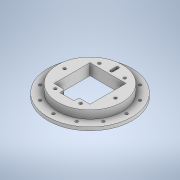
# Autodesk Inventor part: Chasis
Saved by Autodesk Inventor 2022 (Build 260153000, 153)
## iProperties
Created: 2022-02-26
Part Number: Chasis
Material: Genérico
Document SubType Name: Modeling
Designer: JK
Density: 1 g/cm^3
Appearance: Valor por defecto
Author: JK
Autodesk Inventor part; units mm, degrees
ref_plane "YZ Plane" through (0, 0, 0) normal (1, 0, 0) x (0, 1, 0)
ref_plane "XZ Plane" through (0, 0, 0) normal (0, 1, 0) x (-1, 0, 0)
ref_plane "XY Plane" through (0, 0, 0) normal (0, 0, 1) x (1, 0, 0)
sketch "Boceto1" plane through (0, 0, 0) normal (0, 1, 0) x (-1, 0, 0)
  line L0 (-21.7, 21.7) -> (21.7, 21.7)
  line L1 (21.7, 21.7) -> (21.7, -21.7)
  line L2 (21.7, -21.7) -> (-21.7, -21.7)
  line L3 (-21.7, -21.7) -> (-21.7, 21.7)
  line L4 (-21.7, 21.7) -> (21.7, -21.7) construction
  line L5 (21.7, 21.7) -> (-21.7, -21.7) construction
  circle A0 centre (0, 0) radius 39
  dimension "d0" = 43.4
  dimension "d1" = 43.4
  dimension "d2" = 78
  constraints: 12 end point, 2 midpoint, 2 parallel, 1 centre point, 1 coincident, 1 horizontal, 1 perpendicular
  measures "d0" distance of L0.end L1.end
  measures "d1" distance of L1.end L2.end
  measures "d2" diameter of A0
extrude "Extrusión1" add sketch "Boceto1" along normal blind 5.63
sketch "Boceto2" plane through (0, 5.63, 0) normal (0, 1, 0) x (1, 0, 0)
  circle A0 centre (-26, -15.0111) radius 2.15
  line L0 (0, 0) -> (-31.4817, 0)
  line L1 (0, 0) -> (-26, -15.0111)
  circle A1 centre (-26, 15.011) radius 2.15
  circle A2 centre (26, -15.0112) radius 2.15
  circle A3 centre (26, 15.0111) radius 2.15
  line L2 (26, 15.0111) -> (-26, -15.0111)
  line L3 (26, -15.0112) -> (-26, 15.011)
  circle A4 centre (0, 0) radius 39 projected
  line L4 (21.7, -21.7) -> (-21.7, -21.7) projected
  line L5 (-21.7, -21.7) -> (-21.7, 21.7) projected
  line L6 (-21.7, 21.7) -> (21.7, 21.7) projected
  line L7 (21.7, 21.7) -> (21.7, -21.7) projected
  dimension "d5" = 4.3
  dimension "d6" = 30
  dimension "d7" = 26
  dimension "d10" = 26
  dimension "d11" = 30
  dimension "d12" = 26
  dimension "d13" = 26
  dimension "d14" = 15.011
  constraints: 8 end point, 4 centre point, 3 equal radius, 1 collinear, 1 horizontal
  measures "d5" diameter of A0
  measures "d6" angle of L0 L1
  measures "d7" horizontal distance of L0.start L1.end
  measures "d10" horizontal distance of L3.end L0.start
  measures "d11" angle of L0 L3
  measures "d12" horizontal distance of L2.start L0.start
  measures "d13" horizontal distance of L0.start L3.start
  measures "d14" vertical distance of L0.start L3.end
extrude "Extrusión2" cut sketch "Boceto2" against normal through all contours A0 | A1 | A2 | A3
sketch "Boceto3" plane through (0, 5.63, 0) normal (0, 1, 0) x (1, 0, 0)
  circle A0 centre (-26, 15.011) radius 2.15 projected
  circle A1 centre (-26, 15.011) radius 4.3
  line L0 (-21.7, -21.7) -> (-21.7, 21.7) projected
  circle A2 centre (26, 15.0111) radius 2.15 projected
  circle A3 centre (26, 15.0111) radius 4.3
  line L1 (21.7, 21.7) -> (21.7, -21.7) projected
  circle A4 centre (26, -15.0112) radius 2.15 projected
  circle A5 centre (26, -15.0112) radius 4.3
  circle A6 centre (-26, -15.0111) radius 2.15 projected
  circle A7 centre (-26, -15.0111) radius 4.3
  circle A8 centre (26, -15.0112) radius 2.15 projected
  circle A9 centre (26, 15.0111) radius 2.15 projected
  circle A10 centre (-26, -15.0111) radius 2.15 projected
  circle A11 centre (-26, 15.011) radius 2.15 projected
  circle A12 centre (0, 0) radius 39 projected
  line L2 (21.7, -21.7) -> (-21.7, -21.7) projected
  line L3 (-21.7, -21.7) -> (-21.7, 21.7) projected
  line L4 (-21.7, 21.7) -> (21.7, 21.7) projected
  line L5 (21.7, 21.7) -> (21.7, -21.7) projected
  point P0 (-21.7, -15.0111)
  point P1 (-21.7, 15.011)
  point P2 (21.7, 15.0111)
  point P3 (21.7, -15.0112)
  constraints: 4 centre point, 4 coincident, 4 tangent
extrude "Extrusión3" add sketch "Boceto3" along normal blind 4 contours A1 | A3 | A5 | A7 | A12
sketch "Boceto5" plane through (0, 9.63, 0) normal (0, 1, 0) x (1, 0, 0)
  circle A0 centre (-30.6, 0) radius 1.65
  point P0 (0, 0)
  dimension "d24" = 3.3
  dimension "d30" = 30.6
  constraints: 1 centre point
  measures "d24" diameter of A0
  measures "d30" distance of point (0, 0) A0.centre
extrude "Extrusión5" cut sketch "Boceto5" against normal through all
pattern_circular "Patrón circular1" count 6 over 360 about axis through (0, 0, 0) along (0, 1, 0) of "Extrusión5"
sketch "Boceto6" plane through (0, 9.63, 0) normal (0, 1, 0) x (1, 0, 0)
  circle A0 centre (0, 33) radius 1.65
  circle A1 centre (0, 26) radius 1.65
  line L0 (-1.65, 33) -> (1.65, 33)
  line L1 (1.65, 33) -> (1.65, 26)
  line L2 (1.65, 26) -> (-1.65, 26)
  line L3 (-1.65, 26) -> (-1.65, 33)
  point P0 (0, 0)
  point P1 (-1.65, 26)
  dimension "d31" = 3.3
  dimension "d32" = 26
  dimension "d33" = 7
  constraints: 8 end point, 3 vertical, 2 parallel, 1 horizontal, 1 perpendicular, 6 other
  measures "d32" distance of point (0, 0) point (0, 26)
  measures "d33" distance of L0.end L1.end
extrude "Extrusión6" cut sketch "Boceto6" against normal blind 10
sketch "Boceto7" plane through (0, 0, 0) normal (0, -1, 0) x (1, 0, 0)
  line L0 (21.7, 21.7) -> (-21.7, 21.7) projected
  line L1 (8.5, 27.7) -> (-8.5, 27.7)
  line L2 (-8.5, 27.7) -> (-8.5, 21.7)
  line L3 (-8.5, 21.7) -> (8.5, 21.7)
  line L4 (8.5, 21.7) -> (8.5, 27.7)
  point P0 (0, 0)
  dimension "d36" = 8.5
  dimension "d37" = 6
  dimension "d38" = 17
  constraints: 8 end point, 2 parallel, 1 horizontal, 1 perpendicular, 1 point on line
  measures "d36" distance from line of point (0, 0) L4
  measures "d37" distance between parallel lines of L0 L1
  measures "d38" distance between parallel lines of L4 L2
extrude "Extrusión7" cut sketch "Boceto7" against normal through all
fillet "Empalme2" radius 2 4 edges at (8.5, 7.63, 21.7) (8.5, 2.815, 21.7) (-8.5, 2.815, 21.7) (-8.5, 7.63, 21.7)
sketch "Boceto8" plane through (0, 0, 0) normal (0, -1, 0) x (1, 0, 0)
  arc A0 (-10.5, 21.7) -> (-8.5, 23.7) centre (-10.5, 23.7) ccw projected
  line L0 (-8.5, 23.7) -> (-8.5, 27.7) projected
  line L1 (-8.5, 27.7) -> (8.5, 27.7) projected
  line L2 (8.5, 27.7) -> (8.5, 23.7) projected
  arc A1 (8.5, 23.7) -> (10.5, 21.7) centre (10.5, 23.7) ccw projected
  line L3 (21.7, 21.7) -> (10.5, 21.7) projected
  line L4 (21.7, -21.7) -> (21.7, 21.7) projected
  line L5 (-21.7, -21.7) -> (21.7, -21.7) projected
  line L6 (-21.7, 21.7) -> (-21.7, -21.7) projected
  line L7 (-10.5, 21.7) -> (-21.7, 21.7) projected
  circle A2 centre (0, 0) radius 39 projected
  circle A3 centre (-26, -15.011) radius 2.15 projected
  circle A4 centre (-26, 15.0111) radius 2.15 projected
  circle A5 centre (26, -15.0111) radius 2.15 projected
  circle A6 centre (26, 15.0112) radius 2.15 projected
  circle A7 centre (-30.6, 0) radius 1.65 projected
  circle A8 centre (-15.3, 26.5004) radius 1.65 projected
  circle A9 centre (15.3, 26.5004) radius 1.65 projected
  circle A10 centre (30.6, 0) radius 1.65 projected
  circle A11 centre (15.3, -26.5004) radius 1.65 projected
  circle A12 centre (-15.3, -26.5004) radius 1.65 projected
  line L8 (-1.65, -33) -> (-1.65, -26) projected
  arc A13 (1.65, -26) -> (-1.65, -26) centre (0, -26) ccw projected
  line L9 (1.65, -26) -> (1.65, -33) projected
  arc A14 (-1.65, -33) -> (1.65, -33) centre (0, -33) ccw projected
  circle A15 centre (0, 0) radius 50.578
  dimension "d42" = 101.156
  constraints: 1 centre point, 1 coincident
  measures "d42" diameter of A15
extrude "Extrusión8" add sketch "Boceto8" along normal blind 4 contours A2 | A15
sketch "Boceto9" plane through (0, 0, 0) normal (0, 1, 0) x (1, 0, 0)
  circle A0 centre (0, -43.944) radius 1.65
  point P0 (0, 0)
  dimension "d45" = 3.3
  dimension "d46" = 43.944
  constraints: 1 centre point
  measures "d45" diameter of A0
  measures "d46" distance of A0.centre point (0, 0)
extrude "Extrusión9" cut sketch "Boceto9" against normal through all
pattern_circular "Patrón circular2" count 12 over 360 about axis through (0, 0, 0) along (0, -1, 0) of "Extrusión9"
sketch "Boceto10" plane through (0, 9.63, 0) normal (0, 1, 0) x (1, 0, 0)
  circle A0 centre (-26, -15.0111) radius 2.15 projected
  circle A1 centre (-26, 15.011) radius 2.15 projected
  circle A2 centre (26, 15.0111) radius 2.15 projected
  circle A3 centre (26, -15.0112) radius 2.15 projected
  point P0 (0, 0)
extrude "Extrusión10" add sketch "Boceto10" against normal up to surface (13.63 mm away)
sketch "Boceto11" plane through (0, -4, 0) normal (0, -1, 0) x (1, 0, 0)
  circle A0 centre (43.944, 0) radius 1.65 projected
  line L0 (46.794, -1.6454) -> (43.944, -3.2909)
  line L1 (43.944, -3.2909) -> (41.094, -1.6454)
  line L2 (41.094, -1.6454) -> (41.094, 1.6454)
  line L3 (41.094, 1.6454) -> (43.944, 3.2909)
  line L4 (43.944, 3.2909) -> (46.794, 1.6454)
  line L5 (46.794, 1.6454) -> (46.794, -1.6454)
  circle A1 centre (43.944, 0) radius 2.85
  point P0 (0, 0)
  dimension "d54" = 5.7
  constraints: 12 end point, 2 coincident, 1 centre point, 1 tangent, 1 vertical alignment, 13 other
  measures "d54" diameter of A1
extrude "Extrusión11" [suppressed]
pattern_circular "Patrón circular3" [suppressed]
sketch "Boceto12" plane through (0, -4, 0) normal (0, -1, 0) x (1, 0, 0)
  circle A0 centre (15.3, -26.5004) radius 1.65 projected
  circle A1 centre (15.3, -26.5004) radius 2.85
  line L0 (12.0098, -26.5696) -> (13.595, -23.6856)
  line L1 (13.595, -23.6856) -> (16.8852, -23.6164)
  line L2 (16.8852, -23.6164) -> (18.5902, -26.4312)
  line L3 (18.5902, -26.4312) -> (17.005, -29.3152)
  line L4 (17.005, -29.3152) -> (13.7148, -29.3843)
  line L5 (13.7148, -29.3843) -> (12.0098, -26.5696)
  point P0 (0, 0)
  dimension "d60" = 5.7
  constraints: 12 end point, 2 coincident, 1 centre point, 1 tangent, 13 other
  measures "d60" diameter of A1
extrude "Extrusión12" cut sketch "Boceto12" against normal blind 3 contours A0 | A1 | A1 L2 L3 | A1 L1 L2 | L3 L4 A1 | A1 L0 L1 | L4 L5 A1 | A1 L5 L0
pattern_circular "Patrón circular4" count 6 over 360 about axis through (0, 0, 0) along (0, -1, 0) of "Extrusión12"
sketch "Boceto4" plane through (0, 5.63, 0) normal (0, 1, 0) x (1, 0, 0)
  line L0 (21.7, -21.7) -> (-21.7, -21.7) projected
  line L1 (-8.5, -21.7) -> (8.5, -21.7)
  line L2 (8.5, -21.7) -> (8.5, -27.7)
  line L3 (8.5, -27.7) -> (-8.5, -27.7)
  line L4 (-8.5, -27.7) -> (-8.5, -21.7)
  point P0 (0, 0)
  dimension "d18" = 6
  dimension "d19" = 17
  dimension "d20" = 8.5
  constraints: 8 end point, 2 parallel, 1 horizontal, 1 perpendicular, 1 point on line
  measures "d18" distance between parallel lines of L0 L3
  measures "d19" distance between parallel lines of L2 L4
  measures "d20" distance from line of point (0, 0) L4
